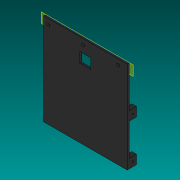
# Autodesk Inventor part: Before
Saved by Autodesk Inventor 2019 (Build 230136000, 136)
## iProperties
Created: 2024-12-30
Part Number: Before
Material: Nylon 6/6
Document SubType Name: Modeling
Designer: Familia CS
Density: 1.13 g/cm^3
Appearance: Black Cast
Author: Familia CS
Autodesk Inventor part; units mm, degrees
ref_plane "YZ Plane" through (0, 0, 0) normal (1, 0, 0) x (0, 1, 0)
ref_plane "XZ Plane" through (0, 0, 0) normal (0, 1, 0) x (-1, 0, 0)
ref_plane "XY Plane" through (0, 0, 0) normal (0, 0, 1) x (1, 0, 0)
ref_plane "Work Plane1" through (0, 0, 0) normal (0, 0, 1) x (1, 0, 0)
sketch "Sketch1" plane through (0, 0, 0) normal (0, 0, 1) x (1, 0, 0)
  line L0 (0, 2) -> (91, 2) projected
  line L1 (51.2, -11.9194) -> (39.8, -11.9194) projected
  line L2 (39.5, -11.9194) -> (39.5, -22.3444) projected
  line L3 (40.05, -22.8694) -> (50.95, -22.8694) projected
  line L4 (51.5, -11.9194) -> (51.5, -22.3444) projected
  line L5 (39.5, -11.9194) -> (51.5, -11.9194)
  line L6 (51.5, -11.9194) -> (51.5, -22.8694)
  line L7 (51.5, -22.8694) -> (39.5, -22.8694)
  line L8 (39.5, -22.8694) -> (39.5, -11.9194)
  line L9 (0, 2) -> (91, 2)
  line L10 (91, 2) -> (91, -98)
  line L11 (91, -98) -> (0, -98)
  line L12 (0, -98) -> (0, 2)
  circle A0 centre (5, -4) radius 0.75 projected
  circle A1 centre (43, -4) radius 0.75 projected
  circle A2 centre (81, -4) radius 0.75 projected
  circle A3 centre (5, -4) radius 1.75
  circle A4 centre (43, -4) radius 1.75
  circle A5 centre (81, -4) radius 1.75
  point P0 (0, 0)
  dimension "d0" = 91
  dimension "d1" = 100
  dimension "d2" = 1
  dimension "d3" = 1
  dimension "d4" = 1
  constraints: 16 end point, 4 parallel, 3 centre point, 2 horizontal, 2 perpendicular, 1 point on line
  measures "d0" distance of L10.end L11.end
  measures "d1" distance of L9.end L10.end
  measures "d2" radial gap between concentric circles of A0 A3
  measures "d3" radial gap between concentric circles of A1 A4
  measures "d4" radial gap between concentric circles of A2 A5
extrude "Extrusion1" add sketch "Sketch1" along normal blind 2 contours L0 L10 L11 L12
sketch "Sketch2" plane through (0, 0, 0) normal (0, 0, -1) x (-1, 0, 0)
  line L0 (-91, 2) -> (0, 2) projected
  line L1 (0, 2) -> (-91, 2)
  point P0 (0, 0)
  constraints: 2 end point, 1 horizontal
sketch "Sketch3" plane through (0, 0, 0) normal (0, 0, -1) x (-1, 0, 0)
  point P0 (0, 0)
sketch "Sketch4" plane through (0, -98, 0) normal (-1, 0, 0) x (0, 0, 1)
  line L0 (0, 100) -> (0, 0) projected
  circle A0 centre (-4, 50) radius 0.75
  line L1 (-8, 50) -> (-8, 55)
  line L2 (-8, 55) -> (0, 55)
  line L3 (0, 55) -> (0, 45)
  line L4 (0, 45) -> (-8, 45)
  line L5 (-8, 45) -> (-8, 50)
  point P0 (0, 98)
  dimension "d8" = 1.5
  dimension "d9" = 4
  dimension "d10" = 5
  dimension "d11" = 8
  dimension "d12" = 10
  dimension "d13" = 8
  constraints: 10 end point, 2 perpendicular, 2 point on line, 1 centre point
  measures "d8" diameter of A0
  measures "d9" distance of A0.centre L1.start
  measures "d10" distance of L1.start L1.end
  measures "d11" distance of L1.end L2.end
  measures "d12" distance of L2.end L3.end
  measures "d13" distance of L3.end L4.end
extrude "Extrusion2" add sketch "Sketch4" against normal blind 5
sketch "Sketch5" plane through (0, -98, 2) normal (-1, 0, 0) x (0, 0, 1)
  line L0 (-2, 0) -> (-2, 45) projected
  line L1 (-2, 0) -> (-10, 0)
  line L2 (-10, 0) -> (-10, 10)
  line L3 (-10, 10) -> (-2, 10)
  line L4 (-2, 10) -> (-2, 0)
  circle A0 centre (-6, 5) radius 0.75
  point P0 (-2, 98)
  dimension "d16" = 8
  dimension "d17" = 10
  dimension "d19" = 1.5
  constraints: 8 end point, 2 parallel, 1 centre point, 1 horizontal, 1 perpendicular
  measures "d16" distance of L2.end L3.end
  measures "d17" distance of L1.end L2.end
  measures "d19" diameter of A0
extrude "Extrusion3" add sketch "Sketch5" against normal blind 5
sketch "Sketch6" plane through (0, -98, 2) normal (0, -1, 0) x (1, 0, 0)
  line L0 (5, -10) -> (5, -2) projected
  line L1 (5, -2) -> (15, -2)
  line L2 (15, -2) -> (15, -10)
  line L3 (15, -10) -> (5, -10)
  line L4 (5, -10) -> (5, -2)
  circle A0 centre (10, -6) radius 0.75
  point P0 (0, -2)
  dimension "d22" = 10
  dimension "d23" = 8
  dimension "d25" = 1.5
  constraints: 8 end point, 2 parallel, 1 centre point, 1 horizontal, 1 perpendicular
  measures "d22" distance of L2.end L3.end
  measures "d23" distance of L1.end L2.end
  measures "d25" diameter of A0
extrude "Extrusion4" add sketch "Sketch6" against normal blind 5
sketch "Sketch7" plane through (91, -98, 0) normal (1, 0, 0) x (0, 0, -1)
  circle A0 centre (4, 50) radius 0.75 projected
  circle A1 centre (4, 50) radius 0.75
  line L0 (8, 45) -> (0, 45) projected
  line L1 (0, 55) -> (8, 55) projected
  line L2 (0, 45) -> (8, 45)
  line L3 (8, 45) -> (8, 55)
  line L4 (8, 55) -> (0, 55)
  line L5 (0, 55) -> (0, 45)
  point P0 (0, 98)
  constraints: 8 end point, 2 parallel, 1 centre point, 1 coincident, 1 horizontal, 1 perpendicular
extrude "Extrusion5" add sketch "Sketch7" against normal blind 5
sketch "Sketch8" plane through (91, -98, 2) normal (1, 0, 0) x (0, 0, -1)
  arc A0 (6.75, 5) -> (5.25, 5) centre (6, 5) ccw projected
  circle A1 centre (6, 5) radius 0.75
  line L0 (10, 10) -> (2, 10) projected
  line L1 (2, 0) -> (10, 0) projected
  line L2 (10, 10) -> (2, 10)
  line L3 (2, 10) -> (2, 0)
  line L4 (2, 0) -> (10, 0)
  line L5 (10, 0) -> (10, 10)
  point P0 (2, 98)
  constraints: 8 end point, 2 parallel, 1 centre point, 1 coincident, 1 horizontal, 1 perpendicular
extrude "Extrusion6" add sketch "Sketch8" against normal blind 5
sketch "Sketch9" plane through (0, -98, 2) normal (0, -1, 0) x (1, 0, 0)
  point P0 (0, -2)
sketch "Sketch10" plane through (0, -98, 2) normal (0, -1, 0) x (1, 0, 0)
  line L0 (86, -2) -> (15, -2) projected
  line L1 (86, -2) -> (76, -2)
  line L2 (76, -2) -> (76, -10)
  line L3 (76, -10) -> (86, -10)
  line L4 (86, -10) -> (86, -2)
  circle A0 centre (81, -6) radius 0.75
  point P0 (0, -2)
  dimension "d32" = 10
  dimension "d33" = 8
  dimension "d35" = 1.5
  constraints: 8 end point, 2 parallel, 1 centre point, 1 horizontal, 1 perpendicular
  measures "d32" distance of L3.end L2.end
  measures "d33" distance of L2.end L1.end
  measures "d35" diameter of A0
extrude "Extrusion7" add sketch "Sketch10" against normal blind 5
sketch "Sketch11" plane through (0, -98, 2) normal (0, -1, 0) x (1, 0, 0)
  line L0 (39.5, -2) -> (51.5, -2) projected
  circle A0 centre (45.5, -6) radius 0.75
  line L1 (45.5, -6) -> (45.5, -10)
  line L2 (45.5, -10) -> (40.5, -10)
  line L3 (40.5, -10) -> (40.5, -2)
  line L4 (40.5, -2) -> (50.5, -2)
  line L5 (50.5, -2) -> (50.5, -10)
  line L6 (50.5, -10) -> (45.5, -10)
  point P0 (0, -2)
  dimension "d39" = 1.5
  dimension "d40" = 4
  dimension "d41" = 5
  dimension "d42" = 8
  dimension "d43" = 10
  dimension "d44" = 8
  constraints: 12 end point, 3 point on line, 2 perpendicular, 1 centre point, 1 vertical
  measures "d39" diameter of A0
  measures "d40" distance of L1.start L1.end
  measures "d41" distance of L1.end L2.end
  measures "d42" distance of L2.end L3.end
  measures "d43" distance of L3.end L4.end
  measures "d44" distance of L4.end L5.end
extrude "Extrusion8" add sketch "Sketch11" against normal blind 5
body "Solid1"
